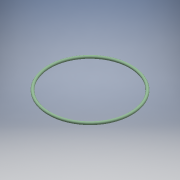
# Autodesk Inventor part: КОДЬЦО 062-066-25 гост 9833
Saved by Autodesk Inventor 2016 (Build 200138000, 138)
## iProperties
Created: 2021-04-24
Part Number: КОДЬЦО 062-066-25 гост 9833
Material: Типовые
Document SubType Name: Modeling
Designer: Лол
Density: 1 g/cm^3
Appearance: По умолчанию
Author: Лол
Autodesk Inventor part; units mm, degrees
ref_plane "YZ Plane" through (0, 0, 0) normal (1, 0, 0) x (0, 1, 0)
ref_plane "XZ Plane" through (0, 0, 0) normal (0, 1, 0) x (-1, 0, 0)
ref_plane "XY Plane" through (0, 0, 0) normal (0, 0, 1) x (1, 0, 0)
sketch "Эскиз1" plane through (0, 0, 0) normal (1, 0, 0) x (0, 1, 0)
  circle A0 centre (37.25, 0) radius 1.25
  line L0 (0, -1.75) -> (0, 1.75) projected
  point P0 (0, 0)
  dimension "d0" = 2.5
  dimension "d1" = 37.25
  constraints: 1 centre point
  measures "d0" diameter of A0
  measures "d1" distance of point (0, 0) A0.centre
revolve "Вращение1" add sketch "Эскиз1" angle 360 about axis through (0, 0, -10) along (0, 0, 1)
